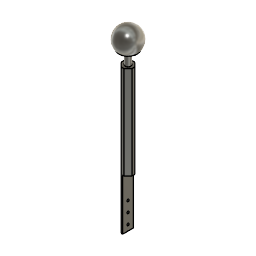
BRAS (Autodesk Fusion 360 design; units mm, degrees)
Autodesk Fusion 360 part; units mm, degrees
sketch "Esquisse1" plane through (0, 0, 0) normal (1, 0, 0) x (0, 1, 0)
sphere "SpherePrimitive1" add diameter 34 placed x (0, 1, 0) y (0, 0, 1) z (1, 0, 0) at (0, 0, 0)
sketch "Esquisse2" plane through (0, 0, 0) normal (0, 0, 1) x (1, 0, 0)
  circle A0 centre (0, 0) radius 2.5
  dimension "d2" = 5
  constraint coincident A0.centre origin
  measures "d2" diameter of A0
extrude "Extrusion1" add sketch "Esquisse2" against normal blind 30
box "BoitePrimitive1" cut length 10 width 10 height 1 placed x (0, 1, 0) y (-1, 0, 0) z (0, 0, 1) at (5, -5, 0)
sketch "Esquisse4" plane through (0, 0, 0) normal (0, 0, 1) x (1, 0, 0)
box "BoitePrimitive2" add length 10 width 10 height 188.75 placed x (0, 1, 0) y (1, 0, 0) z (0, 0, -1) at (-5, -5, -30)
sketch "Esquisse6" plane through (0, 0, -218.75) normal (0, 0, -1) x (1, 0, 0)
  line L0 (-5, -5) -> (5, -5)
  line L1 (5, -5) -> (5, 5)
  line L2 (5, 5) -> (-5, 5)
  line L3 (-5, 5) -> (-5, -5)
extrude "Extrusion2" add sketch "Esquisse6" against normal blind 17.5
move_face "DécalerLesFaces1" offset -1.307 1 faces at (1.6667, -1.6667, -218.75)
sketch "Esquisse7" plane through (5, 0, 0) normal (1, 0, 0) x (0, 1, 0)
hole "Perçage1" at (5, 0.0021, -198.2029) direction (-1, 0, 0) diameter 3 depth 10 tip angle 118
hole "Perçage2" at (5, -0.0059, -205.3239) direction (-1, 0, 0) diameter 3 depth 10 tip angle 118
hole "Perçage3" at (5, 0.0869, -212.4423) direction (-1, 0, 0) diameter 3 depth 10 tip angle 118
sketch "Esquisse8" plane through (0, -5, 0) normal (0, -1, 0) x (1, 0, 0)
  line L0 (5, -217.443) -> (5, -30)
  line L1 (5, -30) -> (-5, -30)
  line L2 (-5, -30) -> (-5, -217.443)
  line L3 (-5, -217.443) -> (5, -217.443)
  line L4 (5, -217.443) -> (0, -217.443)
  line L5 (0, -217.443) -> (0, -157.443)
  line L6 (0, -157.443) -> (5, -157.443)
  line L7 (5, -157.443) -> (5, -217.443)
  dimension "d30" = 60
  constraint horizontal L4
  constraint vertical L5
  constraint horizontal L6
  constraint vertical L7
  constraint coincident L0.start L3.end
  measures "d30" distance of L0.start L6.end
extrude "Extrusion3" cut sketch "Esquisse8" against normal blind 10 contours L0 L3 L4 L5 L6 L7
move_face "DécalerLesFaces2" offset 1.5 1 faces at (2.4969, -0.1246, -21.2101)
move_face "DécalerLesFaces3" offset 5 1 faces at (0, -5, -72.481)
move_face "DécalerLesFaces4" offset 5 1 faces at (0, 5, -72.481)
move_face "DécalerLesFaces5" offset 5 1 faces at (-5, -0.062, -85.5716)
move_face "DécalerLesFaces6" offset 5 1 faces at (5, 3.3333, -114.962)
move_face "DécalerLesFaces7" offset -2.5 1 faces at (10, 3.3333, -114.962)
move_face "DécalerLesFaces8" offset -2.5 1 faces at (-0.8333, -10, -72.481)
move_face "DécalerLesFaces9" offset -2.5 1 faces at (-0.8333, 10, -72.481)
move_face "DécalerLesFaces10" offset -2.5 1 faces at (-10, 0.0007, -85.5676)
sketch "Esquisse9" plane through (0, 0, 0) normal (1, 0, 0) x (0, 1, 0)
  circle A0 centre (-0.0059, -205.3239) radius 1.5
  circle A1 centre (-0.0059, -205.3239) radius 1.5
  circle A2 centre (-0.0059, -191.0859) radius 1.5
  dimension "d42" = 3
  dimension "d43" = 3
  constraint concentric A0 A1
  measures "d42" diameter of A0
  measures "d43" diameter of A2
move_face "DécalerLesFaces11" offset 10 1 faces at (-5, 2.5, -217.443)
hole "Perçage4" at (0, -0.0059, -191.0859) direction (-1, 0, 0) diameter 3 depth 10 tip angle 118
sketch "Esquisse10" plane through (0, 0, 0) normal (1, 0, 0) x (0, 1, 0)
  circle A0 centre (-0.0059, -205.3239) radius 1.5
  circle A1 centre (-0.0059, -205.3239) radius 1.5
  circle A2 centre (-0.0059, -219.5619) radius 1.5
  dimension "d48" = 3
  dimension "d49" = 3
  constraint concentric A0 A1
  measures "d48" diameter of A0
  measures "d49" diameter of A2
hole "Perçage5" at (0, -0.0059, -219.5619) direction (-1, 0, 0) diameter 3 depth 10 tip angle 118
delete_face "DeleteFace1" 1 faces at (-5, -1.2479, -211.758)
delete_face "DeleteFace2" 1 faces at (-5, -1.3327, -197.5186)
chamfer "Chanfrein1" distance 5.5 angle 45 1 edges at (7.5, -7.5, -93.7215)
chamfer "Chanfrein2" distance 5.5 angle 45 1 edges at (7.5, 7.5, -93.7215)
chamfer "Chanfrein3" distance 5.5 angle 45 1 edges at (-7.5, 7.5, -128.7215)
chamfer "Chanfrein4" distance 5.5 angle 45 1 edges at (-7.5, -7.5, -128.7215)
chamfer "Chanfrein5" distance 10 angle 45 1 faces at (13.5236, 2.3846, -10.0213)
sketch "Esquisse11" plane through (0, 0, -30) normal (0, 0, 1) x (-1, 0, 0)
  line L0 (7.5, 2) -> (2, 7.5)
  line L1 (2, 7.5) -> (-2, 7.5)
  line L2 (-2, 7.5) -> (-7.5, 2)
  line L3 (-7.5, 2) -> (-7.5, -2)
  line L4 (-7.5, -2) -> (-2, -7.5)
  line L5 (-2, -7.5) -> (2, -7.5)
  line L6 (2, -7.5) -> (7.5, -2)
  line L7 (7.5, -2) -> (7.5, 2)
  circle A0 centre (0, 0) radius 4
  circle A1 centre (0, 0) radius 30.0923
  circle A2 centre (0, 0) radius 4
  constraint concentric A0 A1
  constraint concentric A1 A2
extrude "Extrusion4" cut sketch "Esquisse11" along normal blind 18.6 contours L0 L1 L2 L3 L4 L5 L6 L7 | A1
equation "d12 = 200 mm - 30 mm + 18.75 mm"
equation "d15 = -202.374 mm - 20 mm - 12.626 mm + 17.5 mm + 200 mm"
